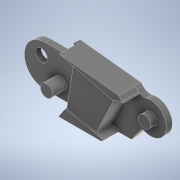
# Autodesk Inventor part: Pieza2
Saved by Autodesk Inventor 2022 (Build 260153000, 153)
## iProperties
Created: 2022-11-04
Part Number: Pieza2
Material: Resina acetálica, negra
Document SubType Name: Modeling
Designer: Mauricio Guerrero
Density: 1.425 g/cm^3
Appearance: Suave - Negro
Author: Mauricio Guerrero
## iProperties of the stored document Pieza2_3DPrint.ipt
Created: 2022-11-06
Part Number: Pieza2_3DPrint
Material: Genérico
Document SubType Name: Modeling
Designer: Mauricio Guerrero
Density: 1 g/cm^3
Appearance: Valor por defecto
Author: Mauricio Guerrero
Autodesk Inventor part; units mm, degrees
ref_plane "YZ Plane" through (0, 0, 0) normal (1, 0, 0) x (0, 1, 0)
ref_plane "XZ Plane" through (0, 0, 0) normal (0, 1, 0) x (-1, 0, 0)
ref_plane "XY Plane" through (0, 0, 0) normal (0, 0, 1) x (1, 0, 0)
sketch "Boceto1" plane through (0, 0, 0) normal (0, 0, 1) x (1, 0, 0)
  circle A0 centre (1.6193, -0.0917) radius 1.25
  circle A1 centre (5.5, -3.0198) radius 1.25
  circle A2 centre (24, -0.0198) radius 1.25
  arc A3 (23.0586, -3.0782) -> (23.1969, 3.0777) centre (24, -0.0198) ccw
  line L0 (22.2281, -2.8226) -> (23.0586, -3.0782)
  line L1 (20.0701, -5.7575) -> (22.2281, -2.8226)
  line L2 (8.358, 5.473) -> (10.9932, 5.5802) construction
  line L3 (8.2096, 5.3474) -> (8.358, 5.473)
  line L4 (21.1684, 3.7215) -> (20.8396, 4.1099)
  line L5 (20.8396, 4.1099) -> (8.358, 5.473)
  arc A4 (21.1684, 3.7215) -> (23.1969, 3.0777) centre (22.6949, 5.0137) ccw
  line L6 (6.8396, 2.5802) -> (2.3489, 2.5802)
  line L7 (20.0701, -5.7575) -> (2.3489, -5.7575)
  arc A5 (2.3489, 2.5802) -> (2.3489, -5.7575) centre (2.3489, -1.5887) ccw
  line L8 (8.358, 3.2519) -> (8.3004, 3.1922)
  line L9 (6.8605, 2.5802) -> (6.7932, 2.5802)
  arc A6 (8.358, 3.2519) -> (8.2096, 5.3474) centre (6.7321, 4.1898) ccw
  arc A7 (6.8605, 2.5802) -> (8.3004, 3.1922) centre (6.8605, 4.5802) ccw
  point P0 (21.1252, -5.0888)
  point P1 (22.1345, 2.5802)
  point P2 (7.7105, 2.5802)
  dimension "d1" = 2.5
  dimension "d33" = 2
  constraints: 20 end point, 11 point on circle, 8 centre point, 4 point on line, 4 tangent, 2 coincident, 2 horizontal
  measures "d1" diameter of A1
  measures "d33" radius of A7
extrude "Extrusión1" add sketch "Boceto1" along normal blind 1.2
sketch "Boceto2" plane through (0, 0, 1.2) normal (0, 0, 1) x (1, 0, 0)
  arc A0 (23.0586, -3.0782) -> (23.1969, 3.0777) centre (24, -0.0198) ccw projected
  line L0 (20.8396, 4.1099) -> (8.358, 5.473) projected
  line L1 (8.7666, 5.4284) -> (20.8396, 4.1099)
  line L2 (20.8396, 4.1099) -> (21.4572, 3.3711)
  line L3 (21.4572, 3.3711) -> (21.7914, 3.2147)
  line L4 (8.7666, 5.4284) -> (19.5399, 2.598)
  arc A1 (21.7914, 3.2147) -> (19.5399, 2.598) centre (21.6249, -0.5954) ccw
  line L5 (8.5436, -5.7575) -> (9.8539, -3.8256)
  line L6 (9.8539, -3.8256) -> (17.608, -5.2919)
  line L7 (17.3447, -5.7575) -> (8.5436, -5.7575)
  arc A2 (17.608, -5.2919) -> (17.3447, -5.7575) centre (17.7053, -5.6542) ccw
  point P0 (0, 0)
  point P1 (0.0237, -5.8)
  point P2 (24.1345, 2.6)
  constraints: 14 end point, 4 point on circle, 2 centre point, 1 collinear, 1 point on line
extrude "Extrusión2" add sketch "Boceto2" along normal blind 3.4
sketch "Boceto3" plane through (0, 0, 0) normal (0, 0, -1) x (-1, 0, 0)
  circle A0 centre (0, 0) radius 1.2362
  circle A1 centre (-5.5, -3.0198) radius 1.25 projected
  circle A2 centre (-5.5, -3.0198) radius 1.25
  circle A3 centre (-24, -0.0198) radius 1.25 projected
  circle A4 centre (-24, -0.0198) radius 1.25
  constraints: 3 centre point, 3 coincident
extrude "Extrusión3" add sketch "Boceto3" against normal blind 2.5 contours A1 | A3
sketch "Boceto4" plane through (5.5, -3.0198, 2.5) normal (0, 0, 1) x (1, 0, 0)
  circle A0 centre (0, 0) radius 1.25 projected
  circle A1 centre (0, 0) radius 1.25
  point P0 (-5.5, 3.0198)
  constraints: 1 centre point, 1 coincident
extrude "Extrusión4" add sketch "Boceto4" along normal blind 1.5
sketch "Boceto6" plane through (0, 0, 1.2) normal (0, 0, 1) x (1, 0, 0)
  line L0 (9.8539, -3.8256) -> (17.608, -5.2919) projected
  line L1 (9.8539, -3.8256) -> (11.2672, 4.7714)
  line L2 (19.5399, 2.598) -> (8.7666, 5.4284) projected
  line L3 (11.2672, 4.7714) -> (19.5399, 2.598)
  line L4 (19.5399, 2.598) -> (15.9763, -4.9536)
  line L5 (9.8539, -3.8256) -> (8.5436, -5.7575) projected
  line L6 (15.9763, -4.9536) -> (9.8539, -3.8256)
  point P0 (0, 0)
  constraints: 8 end point, 1 collinear
extrude "Extrusión6" add sketch "Boceto6" along normal blind 3
